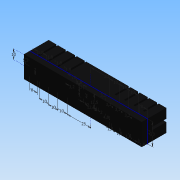
# Autodesk Inventor part: Distance_test_rig
Saved by Autodesk Inventor 2016 (Build 200138000, 138)
## iProperties
Created: 2015-05-18
Part Number: Distance_test_rig
Material: Generic
Document SubType Name: Modeling
Designer: Openlab
Density: 1 g/cm^3
Appearance: Glossy - Black
Author: Openlab
Autodesk Inventor part; units mm, degrees
ref_plane "YZ Plane" through (0, 0, 0) normal (1, 0, 0) x (0, 1, 0)
ref_plane "XZ Plane" through (0, 0, 0) normal (0, 1, 0) x (-1, 0, 0)
ref_plane "XY Plane" through (0, 0, 0) normal (0, 0, 1) x (1, 0, 0)
sketch "Sketch1" plane through (0, 0, 0) normal (0, 1, 0) x (-1, 0, 0)
  line L0 (6.25, 6.25) -> (-6.25, 6.25)
  line L1 (-6.25, 6.25) -> (-6.25, -6.25)
  line L2 (-6.25, -6.25) -> (6.25, -6.25)
  line L3 (6.25, -6.25) -> (6.25, 6.25)
  line L4 (64.8, 11.5) -> (-59.8, 11.5)
  line L5 (-59.8, 11.5) -> (-59.8, -11.5)
  line L6 (-59.8, -11.5) -> (64.8, -11.5)
  line L7 (64.8, -11.5) -> (64.8, 11.5)
  line L8 (70.7232, 0) -> (42.7232, 0) construction
  line L9 (0, 23.25) -> (0, -23.25) construction
  line L10 (-20, -11.5) -> (-20, 11.5)
  line L11 (-30, 11.5) -> (-30, -11.5)
  line L12 (-40, 11.5) -> (-40, -11.5)
  line L13 (-50, 11.5) -> (-50, -11.5)
  line L14 (-51.8, -11.5) -> (-51.8, 11.5)
  line L15 (8.25, -1.5) -> (8.25, -4)
  line L16 (8.25, -1.5) -> (6.25, -1.5)
  line L17 (6.25, 1.5) -> (8.25, 1.5)
  line L18 (-6.25, -1.5) -> (-8.25, -1.5)
  line L19 (-8.25, 1.5) -> (-6.25, 1.5)
  line L20 (55, -6) -> (53.6, -6)
  line L21 (53.6, -6) -> (53.6, 6)
  line L22 (53.6, 6) -> (55, 6)
  line L23 (81.8109, -5) -> (17.0609, -5) construction
  line L24 (81.8109, 5) -> (17.4312, 5) construction
  line L25 (56.8, -6) -> (58.2, -6)
  line L26 (58.2, -6) -> (58.2, -4)
  line L27 (58.2, -4) -> (56.8, -4)
  line L28 (56.8, 4) -> (58.2, 4)
  line L29 (58.2, 4) -> (58.2, 6)
  line L30 (58.2, 6) -> (56.8, 6)
  line L31 (56.8, -11.5) -> (56.8, -6)
  line L32 (55, -6) -> (55, -11.5)
  line L33 (56.8, -4) -> (56.8, 4)
  line L34 (56.8, 6) -> (56.8, 11.5)
  line L35 (55, 11.5) -> (55, 6)
  line L36 (48.2, -6) -> (48.2, -4)
  line L37 (48.2, -4) -> (46.8, -4)
  line L38 (46.8, 6) -> (48.2, 6)
  line L39 (48.2, 6) -> (48.2, 4)
  line L40 (48.2, 4) -> (46.8, 4)
  line L41 (43.6, 6) -> (45, 6)
  line L42 (43.6, -6) -> (45, -6)
  line L43 (46.8, -6) -> (48.2, -6)
  line L44 (46.8, -6) -> (46.8, -11.5)
  line L45 (45, -6) -> (45, -11.5)
  line L46 (46.8, 11.5) -> (46.8, 6)
  line L47 (46.8, 4) -> (46.8, -4)
  line L48 (45, 11.5) -> (45, 6)
  line L49 (38.2, -4) -> (38.2, -6)
  line L50 (38.2, -6) -> (36.8, -6)
  line L51 (35, -6) -> (33.6, -6)
  line L52 (36.8, -4) -> (38.2, -4)
  line L53 (36.8, 4) -> (38.2, 4)
  line L54 (38.2, 4) -> (38.2, 6)
  line L55 (38.2, 6) -> (36.8, 6)
  line L56 (33.6, 6) -> (35, 6)
  line L57 (36.8, -11.5) -> (36.8, -6)
  line L58 (35, -6) -> (35, -11.5)
  line L59 (36.8, -4) -> (36.8, 4)
  line L60 (36.8, 6) -> (36.8, 11.5)
  line L61 (35, 11.5) -> (35, 6)
  line L62 (23.6, 6) -> (23.6, -6)
  line L63 (23.6, -6) -> (25, -6)
  line L64 (26.8, -6) -> (28.2, -6)
  line L65 (28.2, -6) -> (28.2, -4)
  line L66 (28.2, -4) -> (26.8, -4)
  line L67 (26.8, 4) -> (28.2, 4)
  line L68 (28.2, 4) -> (28.2, 6)
  line L69 (28.2, 6) -> (26.8, 6)
  line L70 (26.8, -11.5) -> (26.8, -6)
  line L71 (25, -6) -> (25, -11.5)
  line L72 (26.8, -4) -> (26.8, 4)
  line L73 (26.8, 6) -> (26.8, 11.5)
  line L74 (25, 11.5) -> (25, 6)
  line L75 (8.25, -4) -> (10.05, -4)
  line L76 (10.05, 4) -> (8.25, 4)
  line L77 (8.25, 1.5) -> (8.25, 4)
  line L78 (10.05, -4) -> (10.05, -2.6)
  line L79 (10.05, 2.6) -> (10.05, 4)
  line L80 (-8.25, 4) -> (-10.05, 4)
  line L81 (-10.05, 4) -> (-10.05, 1.5)
  line L82 (-10.05, -1.5) -> (-10.05, -4)
  line L83 (-10.05, -4) -> (-8.25, -4)
  line L84 (-8.25, -4) -> (-8.25, -1.5)
  line L85 (11.8, -2.6) -> (11.8, -6)
  line L86 (11.8, -6) -> (15, -6)
  line L87 (15, -6) -> (15, -2.6)
  line L88 (15, 2.6) -> (15, 6)
  line L89 (15, 6) -> (11.8, 6)
  line L90 (11.8, 6) -> (11.8, 2.6)
  line L91 (-12, -1.5) -> (-12, -6)
  line L92 (-12, -6) -> (-15.2, -6)
  line L93 (-15.2, -6) -> (-15.2, -1.5)
  line L94 (-12, 1.5) -> (-12, 6)
  line L95 (-12, 6) -> (-15.2, 6)
  line L96 (-15.2, 6) -> (-15.2, 1.5)
  line L97 (-10.05, -1.5) -> (-12, -1.5)
  line L98 (-10.05, 1.5) -> (-12, 1.5)
  line L99 (11.8, -2.6) -> (10.05, -2.6)
  line L100 (10.05, 2.6) -> (11.8, 2.6)
  line L101 (56.8, 2.6) -> (64.8, 2.6)
  line L102 (64.8, -2.6) -> (56.8, -2.6)
  line L103 (53.6, -2.6) -> (46.8, -2.6)
  line L104 (46.8, 2.6) -> (53.6, 2.6)
  line L105 (43.6, -2.6) -> (36.8, -2.6)
  line L106 (36.8, 2.6) -> (43.6, 2.6)
  line L107 (33.6, -2.6) -> (26.8, -2.6)
  line L108 (23.6, -2.6) -> (15, -2.6)
  line L109 (15, 2.6) -> (23.6, 2.6)
  line L110 (26.8, 2.6) -> (33.6, 2.6)
  line L111 (-15.2, -1.5) -> (-20, -1.5)
  line L112 (-15.2, 1.5) -> (-20, 1.5)
  line L113 (-51.8, -1.5) -> (-59.8, -1.5)
  line L114 (-51.8, 1.5) -> (-59.8, 1.5)
  line L115 (15, -2.6) -> (15, 2.6)
  line L116 (11.8, -2.6) -> (11.8, 2.6)
  line L117 (10.05, -2.6) -> (10.05, 2.6)
  line L118 (8.25, -1.5) -> (8.25, 1.5)
  line L119 (-10.05, -1.5) -> (-10.05, 1.5)
  line L120 (-12, -1.5) -> (-12, 1.5)
  line L121 (-15.2, -1.5) -> (-15.2, 1.5)
  line L122 (-8.25, 4) -> (-8.25, 1.5)
  line L123 (-8.25, 1.5) -> (-8.25, -1.5)
  line L124 (33.6, -6) -> (33.6, 6)
  line L125 (43.6, 6) -> (43.6, -6)
  line L126 (23.6, 6) -> (25, 6)
  line L127 (-21.8, 6) -> (-23.2, 6)
  line L128 (-23.2, 6) -> (-23.2, 1.5)
  line L129 (-23.2, -1.5) -> (-23.2, -6)
  line L130 (-23.2, -6) -> (-21.8, -6)
  line L131 (-21.8, 11.5) -> (-21.8, 6)
  line L132 (-21.8, -6) -> (-21.8, -11.5)
  line L133 (-23.2, 1.5) -> (-23.2, -1.5)
  line L134 (-23.2, 1.5) -> (-30, 1.5)
  line L135 (-23.2, -1.5) -> (-30, -1.5)
  line L136 (-31.8, 6) -> (-33.2, 6)
  line L137 (-33.2, 6) -> (-33.2, 1.5)
  line L138 (-33.2, -1.5) -> (-33.2, -6)
  line L139 (-33.2, -6) -> (-31.8, -6)
  line L140 (-33.2, -1.5) -> (-33.2, 1.5)
  line L141 (-41.8, 6) -> (-43.2, 6)
  line L142 (-43.2, 6) -> (-43.2, 1.5)
  line L143 (-43.2, -1.5) -> (-43.2, -6)
  line L144 (-41.8, -6) -> (-43.2, -6)
  line L145 (-43.2, 1.5) -> (-43.2, -1.5)
  line L146 (-33.2, 1.5) -> (-40, 1.5)
  line L147 (-33.2, -1.5) -> (-40, -1.5)
  line L148 (-43.2, 1.5) -> (-50, 1.5)
  line L149 (-43.2, -1.5) -> (-50, -1.5)
  line L150 (-41.8, 11.5) -> (-41.8, 6)
  line L151 (-41.8, -6) -> (-41.8, -11.5)
  line L152 (-31.8, 11.5) -> (-31.8, 6)
  line L153 (-31.8, -6) -> (-31.8, -11.5)
  point P0 (0, 0)
  point P1 (0, 0)
  point P2 (0, 0)
  dimension "d0" = 12.5
  dimension "d1" = 12.5
  dimension "d3" = 23
  dimension "d24" = 1.8
  dimension "d62" = 3
  dimension "d96" = 10
  dimension "d97" = 1.8
  dimension "d99" = 1.8
  dimension "d101" = 1.8
  dimension "d103" = 1.8
  dimension "d113" = 8
  dimension "d114" = 1.8
  dimension "d117" = 25
  dimension "d118" = 20
  dimension "d119" = 2
  dimension "d120" = 2
  dimension "d132" = 5.2
  dimension "d133" = 3
  dimension "d135" = 3.2
  dimension "d136" = 3.2
  dimension "d137" = 10
  dimension "d139" = 2
  dimension "d144" = 3.2
  dimension "d145" = 4.8
  dimension "d146" = 10
  dimension "d147" = 10
  dimension "d148" = 10
  dimension "d149" = 1.8
  dimension "d150" = 3.2
  dimension "d151" = 1.8
  dimension "d152" = 1.8
  dimension "d153" = 3.2
  dimension "d154" = 3.2
  dimension "d155" = 10
  dimension "d156" = 10
  dimension "d157" = 10
  dimension "d158" = 8
  dimension "d159" = 8
  constraints: 305 end point, 96 perpendicular, 62 collinear, 46 point on line, 40 vertical, 22 horizontal, 14 equal length, 10 parallel, 2 coincident, 1 midpoint, 56 other
  measures "d0" distance of L2.end L1.end
  measures "d1" distance of L0.end L1.end
  measures "d3" distance of L5.end L5.start
  measures "d24" distance between parallel lines of L14 L13
  measures "d62" distance between parallel lines of L17 L16
  measures "d96" distance between parallel lines of L24 L23
  measures "d97" distance between parallel lines of L35 L34
  measures "d99" distance between parallel lines of L48 L46
  measures "d101" distance between parallel lines of L61 L60
  measures "d103" distance between parallel lines of L74 L73
  measures "d113" distance between parallel lines of L76 L75
  measures "d114" distance between parallel lines of L77 L79
  measures "d117" distance between parallel lines of L9 L71
  measures "d118" distance between parallel lines of L10 L9
  measures "d119" distance between parallel lines of L3 L15
  measures "d120" distance between parallel lines of L84 L1
  measures "d132" distance between parallel lines of L101 L102
  measures "d133" distance between parallel lines of L114 L113
  measures "d135" distance between parallel lines of L62 L72
  measures "d136" distance of L88.end L89.end
  measures "d137" distance between parallel lines of L74 L88
  measures "d139" distance of L25.end L26.end
  measures "d144" distance of L94.end L95.end
  measures "d145" distance between parallel lines of L93 L10
  measures "d146" distance between parallel lines of L58 L71
  measures "d147" distance between parallel lines of L45 L58
  measures "d148" distance between parallel lines of L32 L45
  measures "d149" distance between parallel lines of L10 L132
  measures "d150" distance between parallel lines of L10 L128
  measures "d151" distance between parallel lines of L11 L153
  measures "d152" distance between parallel lines of L12 L151
  measures "d153" distance between parallel lines of L12 L142
  measures "d154" distance between parallel lines of L11 L137
  measures "d155" distance between parallel lines of L11 L10
  measures "d156" distance between parallel lines of L12 L11
  measures "d157" distance between parallel lines of L13 L12
  measures "d158" distance between parallel lines of L7 L31
  measures "d159" distance between parallel lines of L14 L5
extrude "Extrusion10" add sketch "Sketch1" against normal blind 6
extrude "Extrusion16" add sketch "Sketch1" along normal blind 20 contours L0 L1 L19 L122 L80 L81 L98 L94 L95 L96 L112 L10 L4 L74 L126 L62 L109 L88 L89 L90 L100 L79 L76 L77 L17 L3 | L16 L15 L75 L78 L99 L85 L86 L87 L108 L62 L63 L71 L6 L10 L111 L93 L92 L91 L97 L82 L83 L84 L18 L1 L2 L3 | L131 L127 L128 L134 L11 L4 | L6 L11 L135 L129 L130 L132 | L4 L61 L56 L124 L110 L72 L67 L68 L69 L73 | L70 L64 L65 L66 L72 L107 L124 L51 L58 L6 | L152 L136 L137 L146 L12 L4 | L6 L12 L147 L138 L139 L153 | L4 L48 L41 L125 L106 L59 L53 L54 L55 L60 | L57 L50 L49 L52 L59 L105 L125 L42 L45 L6 | L150 L141 L142 L148 L13 L4 | L6 L13 L149 L143 L144 L151 | L4 L35 L22 L21 L104 L47 L40 L39 L38 L46 | L44 L43 L36 L37 L47 L103 L21 L20 L32 L6 | L14 L114 L5 L4 | L6 L5 L113 L14 | L4 L7 L101 L33 L28 L29 L30 L34 | L31 L25 L26 L27 L33 L102 L7 L6
extrude "Extrusion17" add sketch "Sketch1" along normal blind 5 contours L17 L118 L16 L3 | L1 L18 L123 L19 | L100 L116 L99 L117 | L119 L97 L120 L98 | L109 L62 L108 L115 | L121 L111 L10 L112 | L134 L133 L135 L11 | L146 L140 L147 L12 | L124 L107 L72 L110 | L148 L145 L149 L13 | L125 L105 L59 L106 | L14 L113 L5 L114 | L7 L102 L33 L101 | L21 L103 L47 L104
extrude "Extrusion18" add sketch "Sketch1" along normal blind 5 contours L10 L6 L132 L130 L129 L133 L128 L127 L131 L4 | L11 L6 L153 L139 L138 L140 L137 L136 L152 L4 | L12 L6 L151 L144 L143 L145 L142 L141 L150 L4 | L13 L6 L14 L4
body "Solid3"
